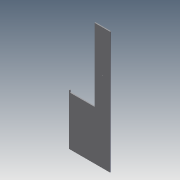
# Autodesk Inventor part: side
Saved by Autodesk Inventor 2011 (Build 150239000, 239)
## iProperties
Created: 2011-10-30
Part Number: side
Document SubType Name: Modeling
Designer: Matthew
Density: 1 g/cm^3
Author: Matthew
Autodesk Inventor part; units mm, degrees
ref_plane "YZ Plane" through (0, 0, 0) normal (1, 0, 0) x (0, 1, 0)
ref_plane "XZ Plane" through (0, 0, 0) normal (0, 1, 0) x (-1, 0, 0)
ref_plane "XY Plane" through (0, 0, 0) normal (0, 0, 1) x (1, 0, 0)
sketch "Sketch1" plane through (0, 0, 0) normal (0, 0, 1) x (1, 0, 0)
  line L0 (-64.9406, 96.6023) -> (189.0594, 96.6023)
  line L1 (189.0594, 96.6023) -> (189.0594, -792.3977)
  line L2 (189.0594, -792.3977) -> (-64.9406, -792.3977)
  line L3 (-64.9406, -792.3977) -> (-64.9406, 96.6023)
  line L4 (-64.9406, 96.6023) -> (87.4594, 96.6023)
  line L5 (87.4594, 96.6023) -> (87.4594, -364.1537)
  line L6 (87.4594, -364.1537) -> (-64.9406, -364.1537)
  line L7 (-64.9406, -364.1537) -> (-64.9406, 96.6023)
  point P0 (0, 0)
  dimension "d0" = 254
  dimension "d1" = 889
  dimension "d2" = 152.4
  dimension "d3" = 460.756
  constraints: 16 end point, 4 parallel, 2 horizontal, 2 perpendicular
  measures "d0" distance of L1.end L2.end
  measures "d1" distance of L0.end L1.end
  measures "d2" distance of L5.end L6.end
  measures "d3" distance of L4.end L5.end
extrude "Extrusion1" add sketch "Sketch1" along normal blind 6.35 contours L0 L1 L2 L3 L6 L5
sketch "Sketch2" plane through (-64.9406, -792.3977, 0) normal (-1, 0, 0) x (0, 0, 1)
  line L0 (6.35, 428.244) -> (0, 428.244) projected
  line L1 (0, 428.244) -> (0, 0) projected
  line L2 (0, 0) -> (6.35, 0) projected
  line L3 (6.35, 0) -> (6.35, 428.244) projected
  point P0 (0, 792.3977)
extrude "Extrusion2" add sketch "Sketch2" along normal blind 6.35
sketch "Sketch3" plane through (0, 0, 6.35) normal (0, 0, 1) x (1, 0, 0)
  line L0 (87.4594, 96.6023) -> (189.0594, 96.6023) projected
  line L1 (87.4594, -364.1537) -> (90.6344, -364.1537)
  line L2 (90.6344, -364.1537) -> (90.6344, 96.6023)
  line L3 (90.6344, 96.6023) -> (87.4594, 96.6023)
  line L4 (87.4594, 96.6023) -> (87.4594, -364.1537)
  point P0 (0, 0)
  dimension "d8" = 3.175
  constraints: 8 end point, 2 parallel, 1 horizontal, 1 perpendicular, 1 point on line
  measures "d8" distance of L3.end L2.end
extrude "Extrusion3" cut sketch "Sketch3" against normal blind 6.35
sketch "Sketch4" plane through (189.0594, 96.6023, 6.35) normal (0, 1, 0) x (1, 0, 0)
  line L0 (-98.425, 6.35) -> (-98.425, 0) projected
  line L1 (-98.425, 0) -> (0, 0) projected
  line L2 (0, 6.35) -> (0, 0) projected
  line L3 (0, 6.35) -> (-98.425, 6.35) projected
  point P0 (-189.0594, 6.35)
extrude "Extrusion4" add sketch "Sketch4" along normal blind 6.35
sketch "Sketch5" plane through (189.0594, 102.9523, 6.35) normal (0, 1, 0) x (1, 0, 0)
  line L0 (-98.425, 6.35) -> (0, 6.35) projected
  line L1 (-98.425, 0) -> (-98.425, 6.35) projected
  line L2 (0, 0) -> (-98.425, 0) projected
  line L3 (0, 6.35) -> (0, 0) projected
  point P0 (-189.0594, 6.35)
extrude "Extrusion5" cut sketch "Sketch5" against normal blind 6.35
sketch "Sketch6" plane through (189.0594, 96.6023, 6.35) normal (0, 1, 0) x (1, 0, 0)
  line L0 (-98.425, 0) -> (-98.425, 6.35) projected
  line L1 (0, 0) -> (-98.425, 0) projected
  line L2 (0, 6.35) -> (0, 0) projected
  line L3 (-98.425, 6.35) -> (0, 6.35) projected
  point P0 (-189.0594, 6.35)
extrude "Extrusion6" add sketch "Sketch6" along normal blind 6.35
sketch "Sketch7" plane through (0, 0, 6.35) normal (0, 0, 1) x (1, 0, 0)
  line L0 (90.6344, -364.1537) -> (-71.2906, -364.1537) projected
  line L1 (-71.2906, -364.1537) -> (-71.2906, -792.3977) projected
  line L2 (189.0594, -792.3977) -> (-71.2906, -792.3977) projected
  line L3 (189.0594, 102.9523) -> (189.0594, -792.3977) projected
  line L4 (189.0594, 102.9523) -> (90.6344, 102.9523) projected
  line L5 (0, -364.1537) -> (0, -688.0037)
  line L6 (0, -688.0037) -> (-71.2906, -688.0037)
  line L7 (0, -688.0037) -> (189.0594, -688.0037)
  point P0 (0, 0)
  dimension "d17" = 323.85
  constraints: 6 end point, 3 point on line, 2 perpendicular, 1 collinear
  measures "d17" distance of L5.start L5.end
extrude "Extrusion7" cut sketch "Sketch7" against normal blind 25.4 contours L7 L3 L2 L1 L6
sketch "Sketch8" plane through (0, 0, 0) normal (0, 0, -1) x (-1, 0, 0)
  line L0 (71.2906, -688.0037) -> (71.2906, -364.1537) projected
  line L1 (-90.6344, -364.1537) -> (71.2906, -364.1537)
  line L2 (71.2906, -364.1537) -> (71.2906, -376.8537)
  line L3 (71.2906, -376.8537) -> (-90.6344, -376.8537)
  line L4 (-90.6344, -376.8537) -> (-90.6344, -364.1537)
  point P0 (0, 0)
  dimension "d20" = 12.7
  constraints: 8 end point, 2 parallel, 1 horizontal, 1 perpendicular, 1 point on line
  measures "d20" distance of L1.end L2.end
extrude "Extrusion8" cut sketch "Sketch8" against normal blind 25.4
sketch "Sketch9" plane through (0, 0, 6.35) normal (0, 0, 1) x (1, 0, 0)
  line L0 (-71.2906, -376.8537) -> (-64.9406, -376.8537)
  line L1 (-64.9406, -376.8537) -> (-64.9406, -364.1537)
  line L2 (-64.9406, -364.1537) -> (-71.2906, -364.1537)
  line L3 (-71.2906, -364.1537) -> (-71.2906, -376.8537)
  point P0 (0, 0)
  dimension "d23" = 6.35
  dimension "d24" = 12.7
  constraints: 8 end point, 2 parallel, 1 horizontal, 1 perpendicular
  measures "d23" distance of L2.end L1.end
  measures "d24" distance of L1.end L0.end
extrude "Extrusion9" add sketch "Sketch9" against normal blind 6.35
sketch "Sketch10" plane through (0, 0, 6.35) normal (0, 0, 1) x (1, 0, 0)
  line L0 (189.0594, 102.9523) -> (189.0594, -688.0037) projected
  line L1 (189.0594, 102.9523) -> (90.6344, 102.9523) projected
  line L2 (90.6344, 102.9523) -> (189.0594, 102.9523)
  line L3 (189.0594, 102.9523) -> (189.0594, 83.9023)
  line L4 (189.0594, 83.9023) -> (90.6344, 83.9023)
  line L5 (90.6344, 83.9023) -> (90.6344, 102.9523)
  point P0 (0, 0)
  dimension "d27" = 19.05
  constraints: 8 end point, 2 parallel, 1 horizontal, 1 perpendicular, 1 point on line
  measures "d27" distance of L2.end L3.end
extrude "Extrusion10" cut sketch "Sketch10" against normal blind 6.35
sketch "Sketch11" plane through (0, 0, 0) normal (0, 0, -1) x (-1, 0, 0)
  line L0 (-189.0594, -688.0037) -> (-189.0594, 83.9023) projected
  line L1 (-189.0594, -688.0037) -> (71.2906, -688.0037) projected
  line L2 (-90.6344, -376.8537) -> (-90.6344, 83.9023) projected
  line L3 (-189.0594, -302.0507) -> (-90.6344, -302.0507)
  line L4 (-139.8469, -302.0507) -> (-139.8469, -688.0037)
  line L5 (-139.8469, -688.0037) -> (-139.8469, -180.0037)
  circle A0 centre (-139.8469, -180.0037) radius 2.3495
  point P0 (0, 0)
  dimension "d30" = 508
  dimension "d31" = 4.699
  constraints: 6 end point, 2 midpoint, 2 perpendicular, 2 point on line, 1 centre point, 1 coincident, 1 parallel
  measures "d30" distance of L4.end L5.end
  measures "d31" diameter of A0
extrude "Extrusion11" cut sketch "Sketch11" against normal blind 25.4 contours A0
sketch "Sketch12" plane through (0, 0, 0) normal (0, 0, -1) x (-1, 0, 0)
  circle A0 centre (-139.8469, -180.0037) radius 2.3495 projected
  line L0 (-90.6344, -376.8537) -> (-90.6344, 83.9023) projected
  line L1 (-139.8469, -180.0037) -> (-139.8469, -410.5087)
  circle A1 centre (-139.8469, -410.5087) radius 2.3495
  point P0 (0, 0)
  dimension "d34" = 230.505
  constraints: 2 end point, 1 centre point, 1 coincident, 1 parallel
  measures "d34" distance of L1.start L1.end
extrude "Extrusion12" cut sketch "Sketch12" against normal blind 25.4 contours A1
body "Solid1"
